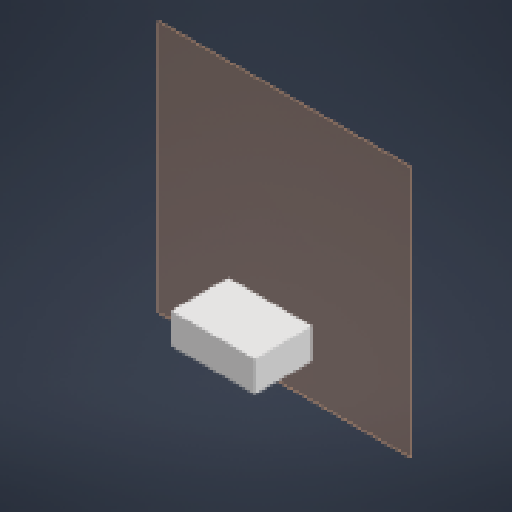
# Autodesk Inventor part: Gref_Sec
Saved by Autodesk Inventor 2024 (Build 280153000, 153)
## iProperties
Created: 2023-04-23
Part Number: Gref_Sec
Material: Genérico
Document SubType Name: Modeling
Designer: javie
Density: 1 g/cm^3
Appearance: Valor por defecto
Author: javie
Autodesk Inventor part; units mm, degrees
ref_plane "YZ Plane" through (0, 0, 0) normal (1, 0, 0) x (0, 1, 0)
ref_plane "XZ Plane" through (0, 0, 0) normal (0, 1, 0) x (-1, 0, 0)
ref_plane "XY Plane" through (0, 0, 0) normal (0, 0, 1) x (1, 0, 0)
ref_plane "Plano de trabajo1" through (0, 0, 0) normal (0, 0, 1) x (1, 0, 0)
sketch "Boceto1" plane through (0, 0, 0) normal (0, 0, 1) x (1, 0, 0)
  line L0 (-1471.3892, -1600.5706) -> (718.6108, -1600.5706)
  line L1 (718.6108, -1600.5706) -> (718.6108, -2400.5706)
  line L2 (718.6108, -2400.5706) -> (-1471.3892, -2400.5706)
  line L3 (-1471.3892, -2400.5706) -> (-1471.3892, -1600.5706)
  line L4 (624.235, -2000.5706) -> (-1372.7834, -2000.5706)
  point P0 (0, 0)
  dimension "d0" = 2190
  dimension "d1" = 800
  dimension "d3" = 400
  constraints: 10 end point, 2 horizontal, 2 parallel, 1 perpendicular
  measures "d0" distance of L1.end L2.end
  measures "d1" distance of L0.end L1.end
  measures "d3" distance between parallel lines of L2 L4
extrude "Extrusión1" add sketch "Boceto1" along normal blind 1150
sketch "Boceto2" plane through (-1471.3892, -2400.5706, 0) normal (0, -1, 0) x (1, 0, 0)
  line L0 (0, 0) -> (2190, 0) projected
  line L1 (0, 0) -> (0, 1150)
  line L2 (0, 0) -> (0, 1150) projected
  line L3 (0, 1150) -> (2190, 1150)
  line L4 (0, 850) -> (2190, 850)
  line L5 (1095, 1150) -> (1095, 0)
  line L6 (2190, 0) -> (2190, 1150) projected
  line L7 (2190, 0) -> (2190, 1150)
  point P0 (1471.3892, 0)
  dimension "d7" = 2190
  dimension "d8" = 1095
  dimension "d9" = 850
  dimension "d11" = 300
  constraints: 10 end point, 2 midpoint, 2 perpendicular, 2 point on line
  measures "d7" distance of L1.end L3.end
  measures "d8" distance between parallel lines of L5 L1
  measures "d9" distance between parallel lines of L4 L0
  measures "d11" distance between parallel lines of L4 L3
sketch "Boceto3" plane through (-1471.3892, -1600.5706, 0) normal (0, 1, 0) x (1, 0, 0)
  line L0 (0, 0) -> (2190, 0) projected
  line L1 (2190, 0) -> (2190, -1150)
  line L2 (2190, 0) -> (2190, -1150) projected
  line L3 (2190, -1150) -> (0, -1150)
  line L4 (0, 0) -> (0, -1150) projected
  line L5 (0, -1150) -> (0, 0)
  line L6 (2190, -850) -> (0, -850)
  line L7 (1095, -1150) -> (1095, 0)
  point P0 (1471.3892, 0)
  dimension "d12" = 1150
  dimension "d13" = 2190
  dimension "d14" = 300
  dimension "d15" = 1095
  constraints: 10 end point, 3 perpendicular, 3 point on line, 2 midpoint
  measures "d12" distance of L0.end L1.end
  measures "d13" distance of L1.end L3.end
  measures "d14" distance between parallel lines of L3 L6
  measures "d15" distance between parallel lines of L4 L7
